Outside Cover Plate (Autodesk Fusion 360 design; units mm, degrees)
Autodesk Fusion 360 part; units mm, degrees
sketch "Sketch1" plane through (0, 0, 0) normal (0, 0, 1) x (1, 0, 0)
  line L0 (0, 0) -> (80, 0)
  line L1 (80, 0) -> (80, 80)
  line L2 (80, 80) -> (0, 80)
  line L3 (0, 80) -> (0, 0)
  circle A0 centre (40, 68.5) radius 1.5
  circle A1 centre (40, 11.5) radius 1.5
  dimension "d1" = 80
  dimension "d2" = 80
  dimension "d3" = 3
  dimension "d4" = 3
  dimension "d5" = 57
  dimension "d6" = 40
  dimension "d7" = 40
  dimension "d8" = 11.5
  constraint horizontal L0
  constraint vertical L1
  constraint horizontal L2
  constraint vertical L3
  constraint coincident L0.start L3.end
  measures "d1" distance of L0.start L0.end
  measures "d2" distance of L0.start L2.end
  measures "d3" diameter of A0
  measures "d4" diameter of A1
  measures "d5" vertical distance of A0.centre A1.centre
  measures "d6" distance of L3 A0.centre
  measures "d7" distance of L3 A1.centre
  measures "d8" distance of L2 A0.centre
extrude "Extrude1" add sketch "Sketch1" along normal blind 2.5
